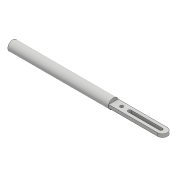
# Autodesk Inventor part: Part3
Saved by Autodesk Inventor 2017 (Build 210142000, 142)
## iProperties
Created: 2019-07-04
Part Number: Part3
Material: Generic
Document SubType Name: Modeling
Designer: Admin
Density: 1 g/cm^3
Appearance: Default
Author: Admin
Autodesk Inventor part; units mm, degrees
ref_plane "XZ Plane" through (0, 0, 0) normal (0, 1, 0) x (-1, 0, 0)
ref_plane "XY Plane" through (0, 0, 0) normal (0, 0, 1) x (1, 0, 0)
sketch "Sketch1" plane through (0, 0, 0) normal (0, 0, 1) x (1, 0, 0)
  line L0 (0, 0) -> (-100, 0) construction
  line L1 (0, 5) -> (-100, 5)
  line L2 (-100, -5) -> (0, -5)
  arc A0 (0, -5) -> (0, 5) centre (0, 0) ccw
  arc A1 (-100, 5) -> (-100, -5) centre (-100, 0) ccw
  line L3 (5, 0) -> (-105, 0) construction
  line L4 (-105, 0) -> (-125, 0)
  circle A2 centre (-125, 0) radius 5
  line L5 (5, 0) -> (-105, 0) construction
  line L6 (5, 15) -> (-125, 15)
  line L7 (-125, -15) -> (5, -15)
  arc A3 (5, -15) -> (5, 15) centre (5, 0) ccw
  line L8 (-125, 15) -> (-710, 15)
  line L9 (-125, -15) -> (-710, -15)
  arc A4 (-710, 15) -> (-710, -15) centre (-710, 0) ccw
  point P0 (-50, 0)
  point P1 (-50, 0)
  point P2 (-50, 0)
  dimension "d0" = 100
  dimension "d1" = 10
  dimension "d3" = 20
  dimension "d6" = 585
  constraints: 26 end point, 10 point on circle, 8 tangent, 5 centre point, 4 horizontal, 3 midpoint, 2 parallel, 1 coincident, 1 collinear
  measures "d0" distance of L0.start L0.end
  measures "d1" diameter of A1
  measures "d3" distance of L3.end L4.end
  measures "d6" distance of L6.end L8.end
extrude "Extrusion1" add sketch "Sketch1" along normal blind 10
ref_plane "Work Plane1" through (-151, 0, 0) normal (1, 0, 0) x (0, 1, 0)
sketch "Sketch2" plane through (-151, 0, 0) normal (1, 0, 0) x (0, 1, 0)
  line L0 (15, 0) -> (15, 10) projected
  circle A0 centre (0, 5) radius 15.8114
  point P0 (0, 0)
  constraints: 3 other
extrude "Extrusion2" add sketch "Sketch2" against normal blind 320
sketch "Sketch3" plane through (0, 0, 10) normal (0, 0, 1) x (1, 0, 0)
  arc A0 (-710, 15) -> (-710, -15) centre (-710, 0) ccw projected
  arc A1 (-710, 15) -> (-710, -15) centre (-710, 0) ccw
  line L0 (-471, 15) -> (-710, 15) projected
  line L1 (-710, -15) -> (-471, -15) projected
  line L2 (-471, 15) -> (-471, -15) projected
  point P0 (0, 0)
  constraints: 2 point on circle, 1 centre point
extrude "Extrusion3" cut sketch "Sketch3" against normal blind 169
hole "Hole1" at (-471, 0, 5) direction (1, 0, 0) diameter 20 depth 305 tip angle 118
body "Solid1"
